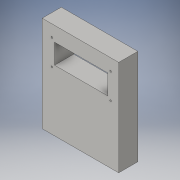
# Autodesk Inventor part: ProtoFront
Saved by Autodesk Inventor 2016 (Build 200138000, 138)
## iProperties
Created: 2018-09-21
Part Number: ProtoFront
Material: Generic
Document SubType Name: Modeling
Designer: student
Density: 1 g/cm^3
Appearance: Default
Author: student
Autodesk Inventor part; units mm, degrees
ref_plane "YZ Plane" through (0, 0, 0) normal (1, 0, 0) x (0, 1, 0)
ref_plane "XZ Plane" through (0, 0, 0) normal (0, 1, 0) x (-1, 0, 0)
ref_plane "XY Plane" through (0, 0, 0) normal (0, 0, 1) x (1, 0, 0)
sketch "Sketch1" plane through (0, 0, 0) normal (0, 0, 1) x (1, 0, 0)
  line L0 (0, 0) -> (101.6, 0)
  line L1 (101.6, 0) -> (101.6, 127)
  line L2 (101.6, 127) -> (0, 127)
  line L3 (0, 127) -> (0, 0)
  line L4 (0, 127) -> (10.668, 127)
  line L5 (101.6, 127) -> (90.932, 127)
  circle A0 centre (90.932, 77.5208) radius 1.1303
  line L6 (87.376, 81.2292) -> (16.4846, 81.2292)
  line L7 (16.4846, 81.2292) -> (16.4846, 107.6706)
  line L8 (16.4846, 107.6706) -> (87.376, 107.6706)
  line L9 (87.376, 107.6706) -> (87.376, 81.2292)
  circle A1 centre (12.9286, 111.379) radius 1.1303
  circle A2 centre (12.9286, 77.5208) radius 1.1303
  circle A3 centre (90.932, 111.379) radius 1.1303
  line L10 (0, 0) -> (12.7, 0)
  line L11 (12.7, 0) -> (12.7, -4.064)
  line L12 (12.7, -4.064) -> (0, -4.064)
  line L13 (0, -4.064) -> (0, 0)
  line L14 (25.4, -4.064) -> (38.1, -4.064)
  line L15 (38.1, -4.064) -> (38.1, 0)
  line L16 (38.1, 0) -> (25.4, 0)
  line L17 (25.4, 0) -> (25.4, -4.064)
  line L18 (50.8, -4.064) -> (63.5, -4.064)
  line L19 (63.5, -4.064) -> (63.5, 0)
  line L20 (63.5, 0) -> (50.8, 0)
  line L21 (50.8, 0) -> (50.8, -4.064)
  line L22 (76.2, -4.064) -> (88.9, -4.064)
  line L23 (88.9, -4.064) -> (88.9, 0)
  line L24 (88.9, 0) -> (76.2, 0)
  line L25 (76.2, 0) -> (76.2, -4.064)
  line L26 (12.7, 127) -> (12.7, 131.064)
  line L27 (12.7, 131.064) -> (0, 131.064)
  line L28 (0, 131.064) -> (0, 127)
  line L29 (25.4, 131.064) -> (38.1, 131.064)
  line L30 (38.1, 131.064) -> (38.1, 127)
  line L31 (25.4, 127) -> (25.4, 131.064)
  line L32 (50.8, 131.064) -> (63.5, 131.064)
  line L33 (63.5, 131.064) -> (63.5, 127)
  line L34 (50.8, 127) -> (50.8, 131.064)
  line L35 (76.2, 131.064) -> (88.9, 131.064)
  line L36 (88.9, 131.064) -> (88.9, 127)
  line L37 (76.2, 127) -> (76.2, 131.064)
  dimension "d0" = 101.6
  dimension "d1" = 127
  dimension "d2" = 10.668
  dimension "d3" = 10.668
  dimension "d7" = 2.2606
  dimension "d23" = 2.2606
  dimension "d24" = 2.2606
  dimension "d25" = 2.2606
  dimension "d28" = 12.7
  dimension "d29" = 4.064
  dimension "d30" = 12.7
  dimension "d31" = 12.7
  dimension "d32" = 12.7
  dimension "d33" = 12.7
  dimension "d34" = 12.7
  dimension "d35" = 12.7
  constraints: 76 end point, 12 parallel, 6 horizontal, 6 perpendicular, 5 point on line, 4 centre point
  measures "d0" distance of L2.end L1.end
  measures "d1" distance of L1.end L0.end
  measures "d2" distance of L2.end L4.end
  measures "d3" distance of L1.end L5.end
  measures "d7" diameter of A0
  measures "d23" diameter of A1
  measures "d24" diameter of A2
  measures "d25" diameter of A3
  measures "d28" distance of L11.end L12.end
  measures "d29" distance of L10.end L11.end
  measures "d30" distance of L11.end L14.start
  measures "d31" distance of L16.end L15.end
  measures "d32" distance of L14.end L18.start
  measures "d33" distance of L20.end L19.end
  measures "d34" distance of L18.end L22.start
  measures "d35" distance of L24.end L23.end
extrude "Extrusion1" add sketch "Sketch1" along normal blind 25.4 contours L3 L2 L1 L0
body "Solid1"
